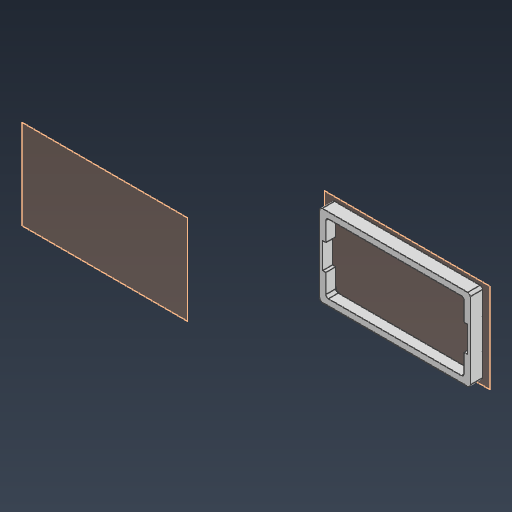
# Autodesk Inventor part: ledy_bateryjki_ramka_check
Saved by Autodesk Inventor 2023 (Build 270158000, 158)
## iProperties
Created: 2025-12-26
Part Number: ledy_bateryjki_ramka_check
Material: Generic
Document SubType Name: Modeling
Designer: szymo
Density: 1 g/cm^3
Appearance: Default
Author: szymo
Autodesk Inventor part; units mm, degrees
ref_plane "YZ Plane" through (0, 0, 0) normal (1, 0, 0) x (0, 1, 0)
ref_plane "XZ Plane" through (0, 0, 0) normal (0, 1, 0) x (-1, 0, 0)
ref_plane "XY Plane" through (0, 0, 0) normal (0, 0, 1) x (1, 0, 0)
ref_plane "Work Plane1" through (0, 0, -12) normal (0, 0, 1) x (1, 0, 0)
ref_plane "Work Plane2" through (101.5856, 16.1884, -33.1044) normal (0, 0, 1) x (1, 0, 0)
sketch "Sketch2" plane through (101.5856, 16.1884, -33.1044) normal (0, 0, 1) x (1, 0, 0)
  line L0 (30.5, -15.5) -> (30.5, 15.5) projected
  arc A0 (30.5, 15.5) -> (29.5, 16.5) centre (29.5, 15.5) ccw projected
  line L1 (29.5, 16.5) -> (-29.5, 16.5) projected
  arc A1 (-29.5, 16.5) -> (-30.5, 15.5) centre (-29.5, 15.5) ccw projected
  line L2 (-30.5, 15.5) -> (-30.5, -15.5) projected
  arc A2 (-30.5, -15.5) -> (-29.5, -16.5) centre (-29.5, -15.5) ccw projected
  line L3 (-29.5, -16.5) -> (29.5, -16.5) projected
  arc A3 (29.5, -16.5) -> (30.5, -15.5) centre (29.5, -15.5) ccw projected
  line L4 (-28, 13) -> (-28, -13) projected
  arc A4 (-27, 14) -> (-28, 13) centre (-27, 13) ccw projected
  line L5 (27, 14) -> (-27, 14) projected
  arc A5 (28, 13) -> (27, 14) centre (27, 13) ccw projected
  line L6 (28, -13) -> (28, 13) projected
  arc A6 (27, -14) -> (28, -13) centre (27, -13) ccw projected
  line L7 (-27, -14) -> (27, -14) projected
  arc A7 (-28, -13) -> (-27, -14) centre (-27, -13) ccw projected
  line L8 (-29.3, 5.25) -> (-29.3, -5.25) projected
  line L9 (-29.3, -5.25) -> (-28, -5.25) projected
  line L10 (-28, 5.25) -> (-28, -5.25) projected
  line L11 (-29.3, 5.25) -> (-28, 5.25) projected
  line L12 (28, 5.25) -> (28, -5.25) projected
  line L13 (28, -5.25) -> (29.3, -5.25) projected
  line L14 (29.3, 5.25) -> (29.3, -5.25) projected
  line L15 (28, 5.25) -> (29.3, 5.25) projected
  point P0 (-101.5856, -16.1884)
extrude "Extrusion2" add sketch "Sketch2" along normal blind 5
chamfer "Chamfer2" distance 1 angle 45 16 edges at (101.5856, 30.1884, -33.1044) (129.2927, 29.8955, -33.1044) (129.5856, 25.3134, -33.1044) (73.8785, 29.8955, -33.1044) (73.5856, 25.3134, -33.1044) (101.5856, 2.1884, -33.1044) (73.8785, 2.4813, -33.1044) (73.5856, 7.0634, -33.1044) (129.2927, 2.4813, -33.1044) (129.5856, 7.0634, -33.1044) (130.2356, 21.4384, -33.1044) (130.2356, 10.9384, -33.1044) (130.8856, 16.1884, -33.1044) (72.9356, 21.4384, -33.1044) (72.2856, 16.1884, -33.1044) (72.9356, 10.9384, -33.1044)
body "Solid2"
